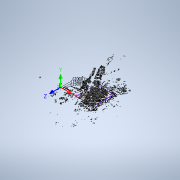
# Autodesk Inventor part: leonOSM
Saved by Autodesk Inventor 2021 (Build 250183000, 183)
## iProperties
Created: 2021-06-19
Part Number: leonOSM
Material: Genérico
Document SubType Name: Modeling
Designer: luise
Density: 1 g/cm^3
Appearance: Valor por defecto
Author: luise
Autodesk Inventor part; units mm, degrees
ref_plane "YZ Plane" through (0, 0, 0) normal (1, 0, 0) x (0, 1, 0)
ref_plane "XZ Plane" through (0, 0, 0) normal (0, 1, 0) x (-1, 0, 0)
ref_plane "XY Plane" through (0, 0, 0) normal (0, 0, 1) x (1, 0, 0)
sketch "Boceto1" plane through (0, 0, 0) normal (0, 1, 0) x (-1, 0, 0)
  line L0 (-1500000, -2000000) -> (-3200000, -2000000)
  line L1 (-3200000, -2000000) -> (-3200000, 0)
  line L2 (-3200000, 0) -> (-1500000, 0)
  line L3 (-1500000, 0) -> (-1500000, -2000000)
  point P0 (0, 0)
  dimension "d7" = 1700000
  dimension "d9" = 2000000
  constraints: 8 end point, 2 parallel, 1 horizontal, 1 perpendicular
  measures "d7" distance between parallel lines of L1 L3
  measures "d9" distance between parallel lines of L2 L0
extrude "Extrusión1" add sketch "Boceto1" against normal blind 1000
sketch "Boceto3" plane through (0, 0, 0) normal (0, 1, 0) x (1, 0, 0)
  line L0 (1500000, 0) -> (3200000, 0) projected
  line L1 (3200000, 0) -> (3200000, 2000000) projected
  line L2 (3200000, 2000000) -> (1500000, 2000000) projected
  line L3 (1500000, 2000000) -> (1500000, 0) projected
  line L4 (3200000, 0) -> (1500000, 0) projected
  line L5 (1500000, 0) -> (1500000, 2000000) projected
  line L6 (3200000, 2000000) -> (3200000, 0) projected
  line L7 (1500000, 2000000) -> (2350000, 2000000)
  line L8 (2350000, 2000000) -> (2350000, 1000000)
  line L9 (2350000, 1000000) -> (1500000, 1000000)
  line L10 (1500000, 1000000) -> (1500000, 2000000)
  line L11 (2350000, 1000000) -> (3200000, 1000000)
  line L12 (3200000, 1000000) -> (3200000, 2000000)
  line L13 (3200000, 2000000) -> (2350000, 2000000)
  line L14 (2350000, 2000000) -> (2350000, 1000000)
  line L15 (2350000, 1000000) -> (1500000, 1000000)
  line L16 (1500000, 1000000) -> (1500000, 0)
  line L17 (1500000, 0) -> (2350000, 0)
  line L18 (2350000, 0) -> (2350000, 1000000)
  line L19 (2350000, 1000000) -> (3200000, 1000000)
  line L20 (3200000, 1000000) -> (3200000, 0)
  line L21 (3200000, 0) -> (2350000, 0)
  line L22 (2350000, 0) -> (2350000, 1000000)
  line L23 (1500000, 1500000) -> (2350000, 1500000)
  point P0 (0, 0)
  dimension "d12" = 1000000
  dimension "d13" = 850000
  dimension "d14" = 1500000
  dimension "d15" = 2000000
  dimension "d16" = 1500000
  constraints: 34 end point, 8 parallel, 4 horizontal, 4 perpendicular, 2 midpoint
  measures "d12" distance between parallel lines of L17 L15
  measures "d13" distance between parallel lines of L22 L3
  measures "d14" distance from line of point (0, 0) L3
  measures "d15" distance from line of point (0, 0) L7
  measures "d16" distance between parallel lines of L0 L23
